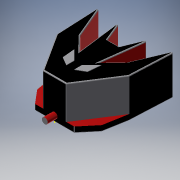
# Autodesk Inventor part: CabezaCarro
Saved by Autodesk Inventor 2017 (Build 210142000, 142)
## iProperties
Part Number: CabezaCarro
Material: Genérico
Document SubType Name: Modeling
Designer: Ghost
Density: 1 g/cm^3
Appearance: Valor por defecto
Author: Ghost
Autodesk Inventor part; units mm, degrees
ref_plane "YZ Plane" through (0, 0, 0) normal (1, 0, 0) x (0, 1, 0)
ref_plane "XZ Plane" through (0, 0, 0) normal (0, 1, 0) x (-1, 0, 0)
ref_plane "XY Plane" through (0, 0, 0) normal (0, 0, 1) x (1, 0, 0)
sketch "Boceto2" plane through (0, 0, 0) normal (0, 0, 1) x (1, 0, 0)
  line L0 (0, 0) -> (-6, 0)
  line L1 (-6, 0) -> (0, 0)
  line L2 (0, 0) -> (6, 0)
  line L3 (-6, 0) -> (-10, 0)
  line L4 (-10, 0) -> (-16.4279, 7.6604)
  line L5 (-16.4279, 7.6604) -> (-18.5117, 19.4781)
  line L6 (-18.5117, 19.4781) -> (-6, 0)
  line L7 (6, 0) -> (10, 0)
  line L8 (10, 0) -> (16.4279, 7.6604)
  line L9 (16.4279, 7.6604) -> (18.5117, 19.4781)
  line L10 (18.5117, 19.4781) -> (6, 0)
  line L11 (-18.5117, 19.4781) -> (-19.6482, 43.4512)
  line L12 (-19.6482, 43.4512) -> (-11.9255, 25.0024)
  line L13 (-11.9255, 25.0024) -> (-5, 17.7887)
  line L14 (-5, 17.7887) -> (-8.1446, 42.5901)
  line L15 (-8.1446, 42.5901) -> (-3, 30)
  line L16 (-3, 30) -> (0, 30)
  line L17 (0, 30) -> (3, 30)
  line L18 (3, 30) -> (8.1446, 42.5901)
  line L19 (8.1446, 42.5901) -> (5, 17.7887)
  line L20 (5, 17.7887) -> (11.9255, 25.0024)
  line L21 (11.9255, 25.0024) -> (19.6482, 43.4512)
  line L22 (19.6482, 43.4512) -> (18.5117, 19.4781)
  point P0 (-1.5, 30)
  dimension "d0" = 6
  dimension "d1" = 6
  dimension "d2" = 4
  dimension "d3" = 130
  dimension "d4" = 150
  dimension "d5" = 12
  dimension "d6" = 10
  dimension "d7" = 130
  dimension "d8" = 24
  dimension "d9" = 20
  dimension "d10" = 25
  dimension "d11" = 20
  dimension "d12" = 10
  dimension "d13" = 150
  dimension "d14" = 15
  dimension "d15" = 3
  dimension "d16" = 30
  dimension "d17" = 10
  constraints: 46 end point, 10 equal length, 5 horizontal alignment, 4 horizontal, 1 midpoint, 1 vertical alignment
  measures "d0" distance of L0.start L0.end
  measures "d1" distance of L0.start L2.end
  measures "d2" distance of L0.end L3.end
  measures "d3" angle of L4 L3
  measures "d4" angle of L4 L5
  measures "d5" distance of L4.end L5.end
  measures "d6" distance of L3.end L4.end
  measures "d7" angle of L8 L7
  measures "d8" distance of L5.end L11.end
  measures "d9" angle of L12 L11
  measures "d10" distance of L13.end L14.end
  measures "d11" distance of L11.end L12.end
  measures "d12" distance of L12.end L13.end
  measures "d13" angle of L22 L10
  measures "d14" angle of L15 L14
  measures "d15" distance of L16.end L17.end
  measures "d16" distance of L0.start L16.end
  measures "d17" distance of L19.end L13.end
extrude "Extrusión1" add sketch "Boceto2" along normal blind 3 contours L3 L4 L5 L6 | L10 L9 L8 L7
extrude "Extrusión2" add sketch "Boceto2" along normal blind 20 contours L0 L6 L11 L12 L13 L14 L15 L16 L17 L18 L19 L20 L21 L22 L10 L2
sketch "Boceto3" plane through (0, 0, 20) normal (0, 0, 1) x (1, 0, 0)
  line L0 (-2, 8) -> (-2, 12)
  line L1 (-2, 12) -> (-6.9268, 16.9726)
  line L2 (-6.9268, 16.9726) -> (-6.3301, 10.5)
  line L3 (-6.3301, 10.5) -> (-2, 8)
  line L4 (2, 8) -> (2, 12)
  line L5 (2, 12) -> (6.9268, 16.9726)
  line L6 (6.9268, 16.9726) -> (6.3301, 10.5)
  line L7 (6.3301, 10.5) -> (2, 8)
  point P0 (0, 0)
  dimension "d22" = 2
  dimension "d23" = 2
  dimension "d24" = 6.5
  dimension "d25" = 7
  dimension "d26" = 4
  dimension "d27" = 60
  dimension "d29" = 5
  dimension "d30" = 8
  constraints: 16 end point, 4 horizontal alignment, 3 equal length, 1 vertical
  measures "d22" horizontal distance of point (0, 0) L0.start
  measures "d23" horizontal distance of point (0, 0) L4.start
  measures "d24" distance of L1.end L2.end
  measures "d25" distance of L0.end L1.end
  measures "d26" distance of L0.start L0.end
  measures "d27" angle of L0 L3
  measures "d29" distance of L2.end L0.start
  measures "d30" vertical distance of point (0, 0) L0.start
extrude "Extrusión3" add sketch "Boceto3" along normal blind 0.25
sketch "Boceto4" plane through (-10, 0, 0) normal (0, -1, 0) x (1, 0, 0)
  point P0 (10, 0)
sketch "Boceto5" plane through (-10, 0, 0) normal (0, -1, 0) x (1, 0, 0)
  point P0 (10, 0)
sketch "Boceto6" plane through (-10, 0, 0) normal (0, -1, 0) x (1, 0, 0)
  circle A0 centre (10, 3) radius 1.5
  line L0 (4, 3) -> (4, 20) projected
  point P0 (10, 0)
  dimension "d33" = 3
  dimension "d34" = 3
  dimension "d35" = 6
  constraints: 1 centre point
  measures "d33" diameter of A0
  measures "d34" distance of point (10, 0) A0.centre
  measures "d35" distance from line of A0.centre L0
extrude "Extrusión4" add sketch "Boceto6" along normal blind 5
sketch "Boceto7" plane through (0, 0, 0) normal (0, 0, -1) x (-1, 0, 0)
  circle A0 centre (0, 15) radius 1.5
  line L0 (10, 0) -> (-10, 0) projected
  point P0 (0, 0)
  point P1 (0, 0)
  dimension "d38" = 3
  dimension "d39" = 15
  constraints: 1 centre point, 1 midpoint, 1 vertical alignment
  measures "d38" diameter of A0
  measures "d39" distance of point (0, 0) A0.centre
extrude "Extrusión5" add sketch "Boceto7" along normal blind 10
fillet "Empalme1" radius 0.5 23 edges at (-19.6482, 43.4512, 10) (-8.1446, 42.5901, 10) (8.1446, 42.5901, 10) (19.6482, 43.4512, 10) (15.7869, 34.2268, 20) (8.4627, 21.3955, 20) (6.5723, 30.1894, 20) (5.5723, 36.2951, 20) (0, 30, 20) (-5.5723, 36.2951, 20) (-6.5723, 30.1894, 20) (-8.4627, 21.3955, 20) (-15.7869, 34.2268, 20) (-19.0799, 31.4647, 20) (-12.2558, 9.7391, 20) (12.2558, 9.7391, 20) (19.0799, 31.4647, 20) (19.0799, 31.4647, 0) (17.4698, 13.5693, 0) (13.2139, 3.8302, 0) (-13.2139, 3.8302, 0) (-17.4698, 13.5693, 0) (-18.5117, 19.4781, 11.5)
fillet "Empalme2" radius 0.5 15 edges at (-16.2905, 7.7245, 0.1464) (-16.4279, 7.6604, 1.75) (-17.467, 13.5536, 3) (-9.8088, 0, 0.1464) (0, 0, 0) (9.8088, 0, 0.1464) (10, 0, 1.75) (-10, 0, 1.75) (-5.8259, 0, 19.8536) (0, 0, 20) (5.8259, 0, 19.8536) (6, 0, 11.25) (-6, 0, 11.25) (18.3672, 19.5243, 19.8536) (18.5117, 19.4781, 11.25)
